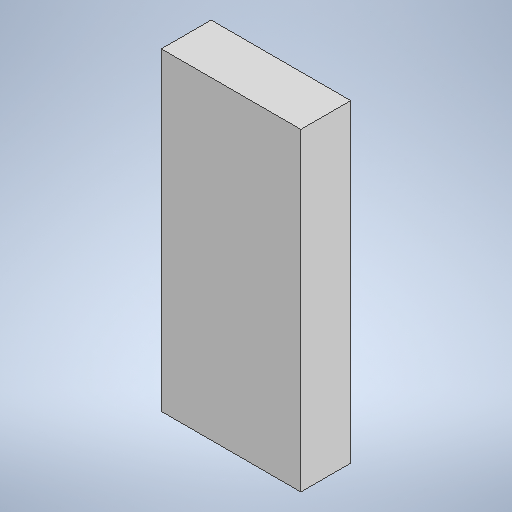
# Autodesk Inventor part: board
Saved by Autodesk Inventor 2026.1 (Build 301233020, 233B)
## iProperties
Created: 2026-02-05
Part Number: board
Material: 一般
Document SubType Name: Modeling
Designer: hibik
Density: 1 g/cm^3
Appearance: 既定
Author: hibik
Autodesk Inventor part; units mm, degrees
ref_plane "YZ Plane" through (0, 0, 0) normal (1, 0, 0) x (0, 1, 0)
ref_plane "XZ Plane" through (0, 0, 0) normal (0, 1, 0) x (-1, 0, 0)
ref_plane "XY Plane" through (0, 0, 0) normal (0, 0, 1) x (1, 0, 0)
sketch "スケッチ1" plane through (0, 0, 0) normal (0, 0, 1) x (1, 0, 0)
  line L0 (14, -31.5) -> (-14, -31.5)
  line L1 (-14, -31.5) -> (-14, 31.5)
  line L2 (-14, 31.5) -> (14, 31.5)
  line L3 (14, 31.5) -> (14, -31.5)
  line L4 (14, -31.5) -> (-14, 31.5) construction
  line L5 (-14, -31.5) -> (14, 31.5) construction
  point P0 (0, 0)
  dimension "d0" = 28
  dimension "d1" = 63
  constraints: 12 end point, 2 midpoint, 2 parallel, 1 horizontal, 1 perpendicular
  measures "d0" distance of L1.end L2.end
  measures "d1" distance of L0.end L1.end
extrude "押し出し1" add sketch "スケッチ1" along normal blind 10
